Autodesk Fusion 360 part; units mm, degrees
(part 2 of 2)
sketch "Sketch12" plane through (0, 25.45, 0) normal (0, -1, 0) x (1, 0, 0)
  circle A0 centre (0, 0) radius 1.25
  arc A1 (5.596, 0.8992) -> (5.3157, 1.9663) centre (0, 0) ccw
  line L0 (5.3157, 1.9663) -> (5.195, 2.0088)
  arc A2 (5.195, 2.0088) -> (4.3152, 1.9854) centre (4.7857, 0.845) ccw
  arc A3 (4.3152, 1.9854) -> (3.8756, 2.7463) centre (0, 0) ccw
  arc A4 (3.8756, 2.7463) -> (4.2572, 3.2479) centre (3.082, 3.7461) ccw
  line L1 (4.2572, 3.2479) -> (4.3966, 3.5768)
  arc A5 (4.3966, 3.5768) -> (3.6204, 4.3608) centre (0, 0) ccw
  line L2 (3.6204, 4.3608) -> (3.4946, 4.3372)
  arc A6 (3.4946, 4.3372) -> (2.7443, 3.877) centre (3.722, 3.1247) ccw
  arc A7 (2.7443, 3.877) -> (1.9832, 4.3162) centre (0, 0) ccw
  arc A8 (1.9832, 4.3162) -> (2.0629, 4.9414) centre (0.7961, 4.7853) ccw
  line L3 (2.0629, 4.9414) -> (2.0192, 5.2959)
  arc A9 (2.0192, 5.2959) -> (0.955, 5.5867) centre (0, 0) ccw
  line L4 (0.955, 5.5867) -> (0.8578, 5.5034)
  arc A10 (0.8578, 5.5034) -> (0.4382, 4.7297) centre (1.6611, 4.5671) ccw
  arc A11 (0.4382, 4.7297) -> (-0.4406, 4.7295) centre (0, 0) ccw
  arc A12 (-0.4406, 4.7295) -> (-0.6842, 5.3109) centre (-1.7032, 4.5422) ccw
  line L5 (-0.6842, 5.3109) -> (-0.8992, 5.596)
  arc A13 (-0.8992, 5.596) -> (-1.9663, 5.3157) centre (0, 0) ccw
  line L6 (-1.9663, 5.3157) -> (-2.0088, 5.195)
  arc A14 (-2.0088, 5.195) -> (-1.9854, 4.3152) centre (-0.845, 4.7857) ccw
  arc A15 (-1.9854, 4.3152) -> (-2.7463, 3.8756) centre (0, 0) ccw
  arc A16 (-2.7463, 3.8756) -> (-3.2479, 4.2572) centre (-3.7461, 3.082) ccw
  line L7 (-3.2479, 4.2572) -> (-3.5768, 4.3966)
  arc A17 (-3.5768, 4.3966) -> (-4.3608, 3.6204) centre (0, 0) ccw
  line L8 (-4.3608, 3.6204) -> (-4.3372, 3.4946)
  arc A18 (-4.3372, 3.4946) -> (-3.877, 2.7443) centre (-3.1247, 3.722) ccw
  arc A19 (-3.877, 2.7443) -> (-4.3162, 1.9832) centre (0, 0) ccw
  arc A20 (-4.3162, 1.9832) -> (-4.9414, 2.0629) centre (-4.7853, 0.7961) ccw
  line L9 (-4.9414, 2.0629) -> (-5.2959, 2.0192)
  arc A21 (-5.2959, 2.0192) -> (-5.5867, 0.955) centre (0, 0) ccw
  line L10 (-5.5867, 0.955) -> (-5.5034, 0.8578)
  arc A22 (-5.5034, 0.8578) -> (-4.7297, 0.4382) centre (-4.5671, 1.6611) ccw
  arc A23 (-4.7297, 0.4382) -> (-4.7295, -0.4406) centre (0, 0) ccw
  arc A24 (-4.7295, -0.4406) -> (-5.3109, -0.6842) centre (-4.5422, -1.7032) ccw
  line L11 (-5.3109, -0.6842) -> (-5.596, -0.8992)
  arc A25 (-5.596, -0.8992) -> (-5.3157, -1.9663) centre (0, 0) ccw
  line L12 (-5.3157, -1.9663) -> (-5.195, -2.0088)
  arc A26 (-5.195, -2.0088) -> (-4.3152, -1.9854) centre (-4.7857, -0.845) ccw
  arc A27 (-4.3152, -1.9854) -> (-3.8756, -2.7463) centre (0, 0) ccw
  arc A28 (-3.8756, -2.7463) -> (-4.2572, -3.2479) centre (-3.082, -3.7461) ccw
  line L13 (-4.2572, -3.2479) -> (-4.3966, -3.5768)
  arc A29 (-4.3966, -3.5768) -> (-3.6204, -4.3608) centre (0, 0) ccw
  line L14 (-3.6204, -4.3608) -> (-3.4946, -4.3372)
  arc A30 (-3.4946, -4.3372) -> (-2.7443, -3.877) centre (-3.722, -3.1247) ccw
  arc A31 (-2.7443, -3.877) -> (-1.9832, -4.3162) centre (0, 0) ccw
  arc A32 (-1.9832, -4.3162) -> (-2.0629, -4.9414) centre (-0.7961, -4.7853) ccw
  line L15 (-2.0629, -4.9414) -> (-2.0192, -5.2959)
  arc A33 (-2.0192, -5.2959) -> (-0.955, -5.5867) centre (0, 0) ccw
  line L16 (-0.955, -5.5867) -> (-0.8578, -5.5034)
  arc A34 (-0.8578, -5.5034) -> (-0.4382, -4.7297) centre (-1.6611, -4.5671) ccw
  arc A35 (-0.4382, -4.7297) -> (0.4406, -4.7295) centre (0, 0) ccw
  arc A36 (0.4406, -4.7295) -> (0.6842, -5.3109) centre (1.7032, -4.5422) ccw
  line L17 (0.6842, -5.3109) -> (0.8992, -5.596)
  arc A37 (0.8992, -5.596) -> (1.9663, -5.3157) centre (0, 0) ccw
  line L18 (1.9663, -5.3157) -> (2.0088, -5.195)
  arc A38 (2.0088, -5.195) -> (1.9854, -4.3152) centre (0.845, -4.7857) ccw
  arc A39 (1.9854, -4.3152) -> (2.7463, -3.8756) centre (0, 0) ccw
  arc A40 (2.7463, -3.8756) -> (3.2479, -4.2572) centre (3.7461, -3.082) ccw
  line L19 (3.2479, -4.2572) -> (3.5768, -4.3966)
  arc A41 (3.5768, -4.3966) -> (4.3608, -3.6204) centre (0, 0) ccw
  line L20 (4.3608, -3.6204) -> (4.3372, -3.4946)
  arc A42 (4.3372, -3.4946) -> (3.877, -2.7443) centre (3.1247, -3.722) ccw
  arc A43 (3.877, -2.7443) -> (4.3162, -1.9832) centre (0, 0) ccw
  arc A44 (4.3162, -1.9832) -> (4.9414, -2.0629) centre (4.7853, -0.7961) ccw
  line L21 (4.9414, -2.0629) -> (5.2959, -2.0192)
  arc A45 (5.2959, -2.0192) -> (5.5867, -0.955) centre (0, 0) ccw
  line L22 (5.5867, -0.955) -> (5.5034, -0.8578)
  arc A46 (5.5034, -0.8578) -> (4.7297, -0.4382) centre (4.5671, -1.6611) ccw
  arc A47 (4.7297, -0.4382) -> (4.7295, 0.4406) centre (0, 0) ccw
  arc A48 (4.7295, 0.4406) -> (5.3109, 0.6842) centre (4.5422, 1.7032) ccw
  line L23 (5.3109, 0.6842) -> (5.596, 0.8992)
  circle A49 centre (0, 0) radius 3.75
  circle A50 centre (0, 0) radius 1.5
extrude "Extrude13" cut sketch "Sketch12" against normal blind 1 contours A49 bodies 12
sketch "Sketch13" plane through (0, 35.45, 0) normal (0, 1, 0) x (1, 0, 0)
  circle A0 centre (0, 0) radius 32.5
  circle A1 centre (0, 0) radius 31.251
  line L0 (1.3544, -28.9433) -> (0.9515, -29.9849)
  arc A2 (0.9515, -29.9849) -> (0.7328, -31.2424) centre (3.9943, -31.1619) ccw
  arc A3 (2.4106, -31.1579) -> (2.0669, -29.9287) centre (-0.8426, -31.4049) ccw
  line L1 (1.5616, -28.9329) -> (2.0669, -29.9287)
  arc A4 (1.3544, -28.9433) -> (1.5616, -28.9329) centre (0, 0) ccw
  line L2 (2.4106, -31.1579) -> (2.4106, -31.4)
  line L3 (2.4106, -31.4) -> (0.7, -31.4)
  line L4 (0.7, -31.4) -> (0.7328, -31.2424)
  line L5 (4.2295, -28.6646) -> (3.9323, -29.7412)
  arc A5 (3.9323, -29.7412) -> (3.8399, -31.0142) centre (7.0772, -30.6093) ccw
  line L6 (3.823, -31.1743) -> (3.8399, -31.0142)
  line L7 (5.525, -31.004) -> (3.823, -31.1743)
  line L8 (5.5009, -30.763) -> (5.525, -31.004)
  arc A6 (5.5009, -30.763) -> (5.0365, -29.5742) centre (2.2886, -31.3327) ccw
  line L9 (4.4346, -28.6336) -> (5.0365, -29.5742)
  arc A7 (4.2295, -28.6646) -> (4.4346, -28.6336) centre (0, 0) ccw
  line L10 (7.0626, -28.1011) -> (6.8741, -29.2018)
  arc A8 (6.8741, -29.2018) -> (6.9089, -30.4777) centre (10.0897, -29.7526) ccw
  line L11 (6.9079, -30.6387) -> (6.9089, -30.4777)
  line L12 (8.5846, -30.2998) -> (6.9079, -30.6387)
  line L13 (8.5366, -30.0625) -> (8.5846, -30.2998)
  arc A9 (8.5366, -30.0625) -> (7.9562, -28.9258) centre (5.3969, -30.9491) ccw
  line L14 (7.2636, -28.0498) -> (7.9562, -28.9258)
  arc A10 (7.0626, -28.1011) -> (7.2636, -28.0498) centre (0, 0) ccw
  line L15 (9.8255, -27.2582) -> (9.7475, -28.3723)
  arc A11 (9.7475, -28.3723) -> (9.9091, -29.6384) centre (13.002, -28.6001) ccw
  line L16 (9.9242, -29.7987) -> (9.9091, -29.6384)
  line L17 (11.5588, -29.2945) -> (9.9242, -29.7987)
  line L18 (11.4874, -29.0631) -> (11.5588, -29.2945)
  arc A12 (11.4874, -29.0631) -> (10.7967, -27.9898) centre (8.4516, -30.258) ccw
  line L19 (10.0204, -27.1872) -> (10.7967, -27.9898)
  arc A13 (9.8255, -27.2582) -> (10.0204, -27.1872) centre (0, 0) ccw
  line L20 (12.4907, -26.1445) -> (12.524, -27.2608)
  arc A14 (12.524, -27.2608) -> (12.8109, -28.5045) centre (15.785, -27.1634) ccw
  line L21 (12.8419, -28.6624) -> (12.8109, -28.5045)
  line L22 (14.4181, -27.998) -> (12.8419, -28.6624)
  line L23 (14.3241, -27.7749) -> (14.4181, -27.998)
  arc A15 (14.3241, -27.7749) -> (13.5299, -26.7758) centre (11.4224, -29.2661) ccw
  line L24 (12.6775, -26.0544) -> (13.5299, -26.7758)
  arc A16 (12.4907, -26.1445) -> (12.6775, -26.0544) centre (0, 0) ccw
  line L25 (15.0318, -24.7709) -> (15.1761, -25.8783)
  arc A17 (15.1761, -25.8783) -> (15.5854, -27.0873) centre (18.4112, -25.4568) ccw
  line L26 (15.6319, -27.2414) -> (15.5854, -27.0873)
  line L27 (17.1342, -26.4233) -> (15.6319, -27.2414)
  line L28 (17.0184, -26.2107) -> (17.1342, -26.4233)
  arc A18 (17.0184, -26.2107) -> (16.1287, -25.2956) centre (14.2796, -27.9834) ccw
  line L29 (15.2087, -24.6626) -> (16.1287, -25.2956)
  arc A19 (15.0318, -24.7709) -> (15.2087, -24.6626) centre (0, 0) ccw
  line L30 (17.4234, -23.1511) -> (17.6773, -24.2387)
  arc A20 (17.6773, -24.2387) -> (18.205, -25.4009) centre (20.8544, -23.4971) ccw
  line L31 (18.2666, -25.5496) -> (18.205, -25.4009)
  line L32 (19.68, -24.586) -> (18.2666, -25.5496)
  line L33 (19.5436, -24.3859) -> (19.68, -24.586)
  arc A21 (19.5436, -24.3859) -> (18.5672, -23.564) centre (16.9948, -26.4225) ccw
  line L34 (17.5887, -23.0258) -> (18.5672, -23.564)
  arc A22 (17.4234, -23.1511) -> (17.5887, -23.0258) centre (0, 0) ccw
  line L35 (19.642, -21.3013) -> (20.0028, -22.3581)
  arc A23 (20.0028, -22.3581) -> (20.6436, -23.462) centre (23.0903, -21.3039) ccw
  line L36 (20.7198, -23.6038) -> (20.6436, -23.462)
  line L37 (22.0301, -22.5043) -> (20.7198, -23.6038)
  line L38 (21.8745, -22.3188) -> (22.0301, -22.5043)
  arc A24 (21.8745, -22.3188) -> (20.8211, -21.5982) centre (19.5412, -24.5991) ccw
  line L39 (19.794, -21.1601) -> (20.8211, -21.5982)
  arc A25 (19.642, -21.3013) -> (19.794, -21.1601) centre (0, 0) ccw
  line L40 (21.6653, -19.2397) -> (22.1296, -20.2554)
  arc A26 (22.1296, -20.2554) -> (22.8771, -21.29) centre (25.0967, -18.899) ccw
  line L41 (22.967, -21.4235) -> (22.8771, -21.29)
  line L42 (24.1614, -20.199) -> (22.967, -21.4235)
  line L43 (23.988, -20.0299) -> (24.1614, -20.199)
  arc A27 (23.988, -20.0299) -> (22.8681, -19.4177) centre (21.8934, -22.5312) ccw
  line L44 (21.8025, -19.0841) -> (22.8681, -19.4177)
  arc A28 (21.6653, -19.2397) -> (21.8025, -19.0841) centre (0, 0) ccw
  line L45 (23.4733, -16.9869) -> (24.0364, -17.9513)
  arc A29 (24.0364, -17.9513) -> (24.8832, -18.9064) centre (26.8538, -16.3062) ccw
  line L46 (24.986, -19.0303) -> (24.8832, -18.9064)
  line L47 (26.0525, -17.6929) -> (24.986, -19.0303)
  line L48 (25.8632, -17.542) -> (26.0525, -17.6929)
  arc A30 (25.8632, -17.542) -> (24.6879, -17.0443) centre (24.028, -20.2393) ccw
  line L49 (23.5943, -16.8184) -> (24.6879, -17.0443)
  arc A31 (23.4733, -16.9869) -> (23.5943, -16.8184) centre (0, 0) ccw
  line L50 (25.048, -14.5653) -> (25.7043, -15.4689)
  arc A32 (25.7043, -15.4689) -> (26.642, -16.3349) centre (28.3439, -13.5514) ccw
  line L51 (26.7566, -16.4479) -> (26.642, -16.3349)
  line L52 (27.6847, -15.011) -> (26.7566, -16.4479)
  line L53 (27.4813, -14.8797) -> (27.6847, -15.011)
  arc A33 (27.4813, -14.8797) -> (26.2623, -14.5015) centre (25.9238, -17.7464) ccw
  line L54 (25.1516, -14.3856) -> (26.2623, -14.5015)
  arc A34 (25.048, -14.5653) -> (25.1516, -14.3856) centre (0, 0) ccw
  line L55 (26.3738, -11.999) -> (27.1168, -12.8327)
  arc A35 (27.1168, -12.8327) -> (28.1361, -13.601) centre (29.5523, -10.662) ccw
  line L56 (28.2613, -13.7021) -> (28.1361, -13.601)
  line L57 (29.0417, -12.1799) -> (28.2613, -13.7021)
  line L58 (28.8263, -12.0695) -> (29.0417, -12.1799)
  arc A36 (28.8263, -12.0695) -> (27.5757, -11.8145) centre (27.5619, -15.077) ccw
  line L59 (26.459, -11.8098) -> (27.5757, -11.8145)
  arc A37 (26.3738, -11.999) -> (26.459, -11.8098) centre (0, 0) ccw
  line L60 (27.4374, -9.3134) -> (28.2598, -10.069)
  arc A38 (28.2598, -10.069) -> (29.3505, -10.732) centre (30.4671, -7.6665) ccw
  line L61 (29.4852, -10.8201) -> (29.3505, -10.732)
  line L62 (30.1101, -9.2278) -> (29.4852, -10.8201)
  line L63 (29.8847, -9.1393) -> (30.1101, -9.2278)
  arc A39 (29.8847, -9.1393) -> (28.615, -9.0102) centre (28.9261, -12.2578) ccw
  line L64 (27.5034, -9.1167) -> (28.615, -9.0102)
  arc A40 (27.4374, -9.3134) -> (27.5034, -9.1167) centre (0, 0) ccw
  line L65 (28.2284, -6.5352) -> (29.1219, -7.2052)
  arc A41 (29.1219, -7.2052) -> (30.2732, -7.7563) centre (31.079, -4.5949) ccw
  line L66 (30.416, -7.8306) -> (30.2732, -7.7563)
  line L67 (30.8793, -6.1839) -> (30.416, -7.8306)
  line L68 (30.6462, -6.1183) -> (30.8793, -6.1839)
  arc A42 (30.6462, -6.1183) -> (29.3699, -6.1163) centre (30.0029, -9.3168) ccw
  line L69 (28.2744, -6.3329) -> (29.3699, -6.1163)
  arc A43 (28.2284, -6.5352) -> (28.2744, -6.3329) centre (0, 0) ccw
  line L70 (28.7388, -3.6921) -> (29.6946, -4.2697)
  arc A44 (29.6946, -4.2697) -> (30.895, -4.7035) centre (31.3821, -1.4776) ccw
  line L71 (31.0445, -4.7632) -> (30.895, -4.7035)
  line L72 (31.3416, -3.0786) -> (31.0445, -4.7632)
  line L73 (31.1031, -3.0366) -> (31.3416, -3.0786)
  arc A45 (31.1031, -3.0366) -> (29.8329, -3.1616) centre (30.7814, -6.2831) ccw
  line L74 (28.7645, -3.4862) -> (29.8329, -3.1616)
  arc A46 (28.7388, -3.6921) -> (28.7645, -3.4862) centre (0, 0) ccw
  line L75 (28.9636, -0.8123) -> (29.9722, -1.2919)
  arc A47 (29.9722, -1.2919) -> (31.2098, -1.604) centre (31.3733, 1.6544) ccw
  line L76 (31.3645, -1.6485) -> (31.2098, -1.604)
  line L77 (31.4923, 0.0573) -> (31.3645, -1.6485)
  line L78 (31.2509, 0.0754) -> (31.4923, 0.0573)
  arc A48 (31.2509, 0.0754) -> (29.9995, -0.1755) centre (31.2541, -3.1871) ccw
  line L79 (28.9687, -0.6049) -> (29.9995, -0.1755)
  arc A49 (28.9636, -0.8123) -> (28.9687, -0.6049) centre (0, 0) ccw
  line L80 (28.9006, 2.0756) -> (29.9519, 1.6988)
  arc A50 (29.9519, 1.6988) -> (31.2144, 1.5115) centre (31.0526, 4.77) ccw
  line L81 (31.3728, 1.4826) -> (31.2144, 1.5115)
  line L82 (31.3301, 3.1926) -> (31.3728, 1.4826)
  line L83 (31.0881, 3.1866) -> (31.3301, 3.1926)
  arc A51 (31.0881, 3.1866) -> (29.8679, 2.8124) centre (31.4161, -0.0593) ccw
  line L84 (28.885, 2.2825) -> (29.8679, 2.8124)
  arc A52 (28.9006, 2.0756) -> (28.885, 2.2825) centre (0, 0) ccw
  line L85 (28.5503, 4.9428) -> (29.6339, 4.6726)
  arc A53 (29.6339, 4.6726) -> (30.9088, 4.6119) centre (30.4234, 7.8381) ccw
  line L86 (31.0693, 4.599) -> (30.9088, 4.6119)
  line L87 (30.8566, 6.2963) -> (31.0693, 4.599)
  line L88 (30.6163, 6.2661) -> (30.8566, 6.2963)
  arc A54 (30.6163, 6.2661) -> (29.4394, 5.7723) centre (31.2659, 3.069) ccw
  line L89 (28.5142, 5.1471) -> (29.4394, 5.7723)
  arc A55 (28.5503, 4.9428) -> (28.5142, 5.1471) centre (0, 0) ccw
  line L90 (27.9163, 7.761) -> (29.0214, 7.5999)
  arc A56 (29.0214, 7.5999) -> (30.296, 7.6665) centre (29.4918, 10.8283) ccw
  line L91 (30.457, 7.6696) -> (30.296, 7.6665)
  line L92 (30.0763, 9.3373) -> (30.457, 7.6696)
  line L93 (29.8403, 9.2834) -> (30.0763, 9.3373)
  arc A57 (29.8403, 9.2834) -> (28.7184, 8.6748) centre (30.805, 6.1668) ccw
  line L94 (27.86, 7.9606) -> (28.7184, 8.6748)
  arc A58 (27.9163, 7.761) -> (27.86, 7.9606) centre (0, 0) ccw
  line L95 (27.0048, 10.502) -> (28.1205, 10.4518)
  arc A59 (28.1205, 10.4518) -> (29.3821, 10.6449) centre (28.2671, 13.711) ccw
  line L96 (29.542, 10.664) -> (29.3821, 10.6449)
  line L97 (28.9972, 12.2855) -> (29.542, 10.664)
  line L98 (28.7677, 12.2084) -> (28.9972, 12.2855)
  arc A60 (28.7677, 12.2084) -> (27.712, 11.4911) centre (30.0379, 9.2034) ccw
  line L99 (26.9289, 10.695) -> (27.712, 11.4911)
  arc A61 (27.0048, 10.502) -> (26.9289, 10.695) centre (0, 0) ccw
  line L100 (25.825, 13.1386) -> (26.9401, 13.1997)
  arc A62 (26.9401, 13.1997) -> (28.1762, 13.5176) centre (26.7614, 16.4573) ccw
  line L101 (28.3334, 13.5525) -> (28.1762, 13.5176)
  line L102 (27.6298, 15.1117) -> (28.3334, 13.5525)
  line L103 (27.4092, 15.0121) -> (27.6298, 15.1117)
  arc A63 (27.4092, 15.0121) -> (26.4301, 14.1933) centre (28.9723, 12.1484) ccw
  line L104 (25.7302, 13.3232) -> (26.4301, 14.1933)
  arc A64 (25.825, 13.1386) -> (25.7302, 13.3232) centre (0, 0) ccw
  line L105 (24.3884, 15.6446) -> (25.4919, 15.8165)
  arc A65 (25.4919, 15.8165) -> (26.6903, 16.2558) centre (24.9898, 19.0401) ccw
  line L106 (26.8432, 16.3062) -> (26.6903, 16.2558)
  line L107 (25.9879, 17.7876) -> (26.8432, 16.3062)
  line L108 (25.7782, 17.6666) -> (25.9879, 17.7876)
  arc A66 (25.7782, 17.6666) -> (24.8856, 16.7543) centre (27.6187, 14.9728) ccw
  line L109 (24.2758, 15.8188) -> (24.8856, 16.7543)
  arc A67 (24.3884, 15.6446) -> (24.2758, 15.8188) centre (0, 0) ccw
  line L110 (22.7095, 17.9952) -> (23.7904, 18.2761)
  arc A68 (23.7904, 18.2761) -> (24.9391, 18.8326) centre (22.9699, 21.4337) ccw
  line L111 (25.0862, 18.8979) -> (24.9391, 18.8326)
  line L112 (24.0877, 20.2868) -> (25.0862, 18.8979)
  line L113 (23.8911, 20.1455) -> (24.0877, 20.2868)
  arc A69 (23.8911, 20.1455) -> (23.0937, 19.1489) centre (25.9906, 17.6483) ccw
  line L114 (22.5801, 18.1573) -> (23.0937, 19.1489)
  arc A70 (22.7095, 17.9952) -> (22.5801, 18.1573) centre (0, 0) ccw
  line L115 (20.805, 20.1669) -> (21.8525, 20.554)
  arc A71 (21.8525, 20.554) -> (22.9401, 21.2221) centre (20.7216, 23.6142) ccw
  line L116 (23.0799, 21.3018) -> (22.9401, 21.2221)
  line L117 (21.9481, 22.5843) -> (23.0799, 21.3018)
  line L118 (21.7666, 22.4241) -> (21.9481, 22.5843)
  arc A72 (21.7666, 22.4241) -> (21.0724, 21.3531) centre (24.1043, 20.1484) ccw
  line L119 (20.66, 20.3154) -> (21.0724, 21.3531)
  arc A73 (20.805, 20.1669) -> (20.66, 20.3154) centre (0, 0) ccw
  line L120 (18.6936, 22.1382) -> (19.6974, 22.6277)
  arc A74 (19.6974, 22.6277) -> (20.713, 23.4007) centre (18.2674, 25.5601) ccw
  line L121 (20.8443, 23.4939) -> (20.713, 23.4007)
  line L122 (19.5904, 24.6574) -> (20.8443, 23.4939)
  line L123 (19.4257, 24.48) -> (19.5904, 24.6574)
  arc A75 (19.4257, 24.48) -> (18.8416, 23.3451) centre (21.9784, 22.4483) ccw
  line L124 (18.5346, 22.2715) -> (18.8416, 23.3451)
  arc A76 (18.6936, 22.1382) -> (18.5346, 22.2715) centre (0, 0) ccw
  line L125 (16.3964, 23.8895) -> (17.3465, 24.4765)
  arc A77 (17.3465, 24.4765) -> (18.2801, 25.3468) centre (15.6317, 27.2519) ccw
  line L126 (18.4015, 25.4526) -> (18.2801, 25.3468)
  line L127 (17.0379, 26.4855) -> (18.4015, 25.4526)
  line L128 (16.8917, 26.2925) -> (17.0379, 26.4855)
  arc A78 (16.8917, 26.2925) -> (16.4235, 25.1051) centre (19.634, 24.5251) ccw
  line L129 (16.225, 24.0063) -> (16.4235, 25.1051)
  arc A79 (16.3964, 23.8895) -> (16.225, 24.0063) centre (0, 0) ccw
  line L130 (13.9363, 25.4033) -> (14.8233, 26.082)
  arc A80 (14.8233, 26.082) -> (15.6656, 27.041) centre (12.8406, 28.6729) ccw
  line L131 (15.7758, 27.1583) -> (15.6656, 27.041)
  line L132 (14.3161, 28.0503) -> (15.7758, 27.1583)
  line L133 (14.1899, 27.8437) -> (14.3161, 28.0503)
  arc A81 (14.1899, 27.8437) -> (13.8422, 26.6156) centre (17.0945, 26.3582) ccw
  line L134 (13.7541, 25.5025) -> (13.8422, 26.6156)
  arc A82 (13.9363, 25.4033) -> (13.7541, 25.5025) centre (0, 0) ccw
  line L135 (11.3377, 26.6647) -> (12.1527, 27.4283)
  arc A83 (12.1527, 27.4283) -> (12.8953, 28.4664) centre (9.9219, 29.809) ccw
  line L136 (12.9933, 28.5941) -> (12.8953, 28.4664)
  line L137 (11.4521, 29.3363) -> (12.9933, 28.5941)
  line L138 (11.3471, 29.1182) -> (11.4521, 29.3363)
  arc A84 (11.3471, 29.1182) -> (11.1234, 27.8616) centre (14.3852, 27.9292) ccw
  line L139 (11.1465, 26.7452) -> (11.1234, 27.8616)
  arc A85 (11.3377, 26.6647) -> (11.1465, 26.7452) centre (0, 0) ccw
  line L140 (8.6265, 27.6611) -> (9.3613, 28.502)
  arc A86 (9.3613, 28.502) -> (9.9969, 29.6089) centre (6.9046, 30.6487) ccw
  line L141 (10.0816, 29.7458) -> (9.9969, 29.6089)
  line L142 (8.4742, 30.3308) -> (10.0816, 29.7458)
  line L143 (8.3914, 30.1033) -> (8.4742, 30.3308)
  arc A87 (8.3914, 30.1033) -> (8.294, 28.8307) centre (11.5328, 29.2228) ccw
  line L144 (8.4282, 27.7221) -> (8.294, 28.8307)
  arc A88 (8.6265, 27.6611) -> (8.4282, 27.7221) centre (0, 0) ccw
  line L145 (5.8294, 28.3825) -> (6.4769, 29.2925)
  arc A89 (6.4769, 29.2925) -> (6.9991, 30.4571) centre (3.8186, 31.1839) ccw
  line L146 (7.0698, 30.6018) -> (6.9991, 30.4571)
  line L147 (5.4122, 31.0239) -> (7.0698, 30.6018)
  line L148 (5.3524, 30.7892) -> (5.4122, 31.0239)
  arc A90 (5.3524, 30.7892) -> (5.3822, 29.5133) centre (8.5659, 30.2258) ccw
  line L149 (5.6261, 28.4235) -> (5.3822, 29.5133)
  arc A91 (5.8294, 28.3825) -> (5.6261, 28.4235) centre (0, 0) ccw
  line L150 (2.9745, 28.8219) -> (3.5281, 29.7918)
  arc A92 (3.5281, 29.7918) -> (3.9318, 31.0027) centre (0.6947, 31.4092) ccw
  line L151 (3.9877, 31.1536) -> (3.9318, 31.0027)
  line L152 (2.2963, 31.4086) -> (3.9877, 31.1536)
  line L153 (2.2602, 31.1692) -> (2.2963, 31.4086)
  arc A93 (2.2602, 31.1692) -> (2.4169, 29.9025) centre (5.5138, 30.9285) ccw
  line L154 (2.768, 28.8425) -> (2.4169, 29.9025)
  arc A94 (2.9745, 28.8219) -> (2.768, 28.8425) centre (0, 0) ccw
  line L155 (0.09, 28.9749) -> (0.5443, 29.9951)
  arc A95 (0.5443, 29.9951) -> (0.8254, 31.2401) centre (-2.4361, 31.3223) ccw
  line L156 (0.866, 31.3959) -> (0.8254, 31.2401)
  line L157 (-0.8424, 31.4811) -> (0.866, 31.3959)
  line L158 (-0.8545, 31.2393) -> (-0.8424, 31.4811)
  arc A96 (-0.8545, 31.2393) -> (-0.5725, 29.9945) centre (2.4069, 31.3238) ccw
  line L159 (-0.1175, 28.9748) -> (-0.5725, 29.9945)
  arc A97 (0.09, 28.9749) -> (-0.1175, 28.9748) centre (0, 0) ccw
  line L160 (-2.7955, 28.8398) -> (-2.445, 29.9002)
  arc A98 (-2.445, 29.9002) -> (-2.2892, 31.167) centre (-5.5426, 30.9241) ccw
  line L161 (-2.2643, 31.3261) -> (-2.2892, 31.167)
  line L162 (-3.9727, 31.2408) -> (-2.2643, 31.3261)
  line L163 (-3.9607, 30.999) -> (-3.9727, 31.2408)
  arc A99 (-3.9607, 30.999) -> (-3.5561, 29.7885) centre (-0.7239, 31.4078) ccw
  line L164 (-3.0019, 28.8191) -> (-3.5561, 29.7885)
  arc A100 (-2.7955, 28.8398) -> (-3.0019, 28.8191) centre (0, 0) ccw
  line L165 (-5.6531, 28.4182) -> (-5.4099, 29.5082)
  arc A101 (-5.4099, 29.5082) -> (-5.3811, 30.7842) centre (-8.5941, 30.2185) ccw
  line L166 (-5.3721, 30.945) -> (-5.3811, 30.7842)
  line L167 (-7.0636, 30.69) -> (-5.3721, 30.945)
  line L168 (-7.0275, 30.4506) -> (-7.0636, 30.69)
  arc A102 (-7.0275, 30.4506) -> (-6.5044, 29.2864) centre (-3.8475, 31.1797) ccw
  line L169 (-5.8564, 28.377) -> (-6.5044, 29.2864)
  arc A103 (-5.6531, 28.4182) -> (-5.8564, 28.377) centre (0, 0) ccw
  line L170 (-8.4545, 27.7141) -> (-8.3211, 28.8229)
  arc A104 (-8.3211, 28.8229) -> (-8.4195, 30.0955) centre (-11.5602, 29.2127) ccw
  line L171 (-8.4265, 30.2563) -> (-8.4195, 30.0955)
  line L172 (-10.0842, 29.8342) -> (-8.4265, 30.2563)
  line L173 (-10.0245, 29.5996) -> (-10.0842, 29.8342)
  arc A105 (-10.0245, 29.5996) -> (-9.3881, 28.4932) centre (-6.9329, 30.6416) ccw
  line L174 (-8.6527, 27.6529) -> (-9.3881, 28.4932)
  arc A106 (-8.4545, 27.7141) -> (-8.6527, 27.6529) centre (0, 0) ccw
  line L175 (-11.172, 26.7346) -> (-11.1496, 27.8512)
  arc A107 (-11.1496, 27.8512) -> (-11.3742, 29.1076) centre (-14.4114, 27.9165) ccw
  line L176 (-11.3972, 29.2669) -> (-11.3742, 29.1076)
  line L177 (-13.0046, 28.6819) -> (-11.3972, 29.2669)
  line L178 (-12.9218, 28.4544) -> (-13.0046, 28.6819)
  arc A108 (-12.9218, 28.4544) -> (-12.1785, 27.4169) centre (-9.9494, 29.7991) ccw
  line L179 (-11.3631, 26.6539) -> (-12.1785, 27.4169)
  arc A109 (-11.172, 26.7346) -> (-11.3631, 26.6539) centre (0, 0) ccw
  line L180 (-13.7783, 25.4894) -> (-13.8673, 26.6026)
  arc A110 (-13.8673, 26.6026) -> (-14.2158, 27.8305) centre (-17.1194, 26.3428) ccw
  line L181 (-14.2546, 27.9867) -> (-14.2158, 27.8305)
  line L182 (-15.7958, 27.2445) -> (-14.2546, 27.9867)
  line L183 (-15.6907, 27.0264) -> (-15.7958, 27.2445)
  arc A111 (-15.6907, 27.0264) -> (-14.8478, 26.0681) centre (-12.8669, 28.6604) ccw
  line L184 (-13.9605, 25.3901) -> (-14.8478, 26.0681)
  arc A112 (-13.7783, 25.4894) -> (-13.9605, 25.3901) centre (0, 0) ccw
  line L185 (-16.2478, 23.9908) -> (-16.4471, 25.0897)
  arc A113 (-16.4471, 25.0897) -> (-16.9162, 26.2767) centre (-19.6572, 24.5074) ccw
  line L186 (-16.9704, 26.4283) -> (-16.9162, 26.2767)
  line L187 (-18.43, 25.5364) -> (-16.9704, 26.4283)
  line L188 (-18.3037, 25.3298) -> (-18.43, 25.5364)
  arc A114 (-18.3037, 25.3298) -> (-17.3695, 24.4602) centre (-15.6567, 27.2368) ccw
  line L189 (-16.4191, 23.8739) -> (-17.3695, 24.4602)
  arc A115 (-16.2478, 23.9908) -> (-16.4191, 23.8739) centre (0, 0) ccw
  line L190 (-18.5558, 22.2539) -> (-18.8635, 23.3274)
  arc A116 (-18.8635, 23.3274) -> (-19.4485, 24.4619) centre (-21.9997, 22.4284) ccw
  line L191 (-19.5175, 24.6073) -> (-19.4485, 24.4619)
  line L192 (-20.881, 23.5744) -> (-19.5175, 24.6073)
  line L193 (-20.7348, 23.3815) -> (-20.881, 23.5744)
  arc A117 (-20.7348, 23.3815) -> (-19.7187, 22.6092) centre (-18.2908, 25.5426) ccw
  line L194 (-18.7146, 22.1204) -> (-19.7187, 22.6092)
  arc A118 (-18.5558, 22.2539) -> (-18.7146, 22.1204) centre (0, 0) ccw
  line L195 (-20.6793, 20.2957) -> (-21.0924, 21.3333)
  arc A119 (-21.0924, 21.3333) -> (-21.7874, 22.4039) centre (-24.1235, 20.1265) ccw
  line L196 (-21.8706, 22.5417) -> (-21.7874, 22.4039)
  line L197 (-23.1245, 21.3782) -> (-21.8706, 22.5417)
  line L198 (-22.9598, 21.2007) -> (-23.1245, 21.3782)
  arc A120 (-22.9598, 21.2007) -> (-21.8718, 20.5335) centre (-20.7431, 23.5945) ccw
  line L199 (-20.8241, 20.1471) -> (-21.8718, 20.5335)
  arc A121 (-20.6793, 20.2957) -> (-20.8241, 20.1471) centre (0, 0) ccw
  line L200 (-22.5974, 18.1359) -> (-23.1117, 19.1271)
  arc A122 (-23.1117, 19.1271) -> (-23.9099, 20.1232) centre (-26.0076, 17.6245) ccw
  line L201 (-24.0063, 20.2521) -> (-23.9099, 20.1232)
  line L202 (-25.1382, 18.9695) -> (-24.0063, 20.2521)
  line L203 (-24.9566, 18.8093) -> (-25.1382, 18.9695)
  arc A123 (-24.9566, 18.8093) -> (-23.8076, 18.2537) centre (-22.9893, 21.4119) ccw
  line L204 (-22.7266, 17.9736) -> (-23.8076, 18.2537)
  arc A124 (-22.5974, 18.1359) -> (-22.7266, 17.9736) centre (0, 0) ccw
  line L205 (-24.2908, 15.7958) -> (-24.9013, 16.7309)
  arc A125 (-24.9013, 16.7309) -> (-25.7947, 17.6426) centre (-27.6332, 14.9474) ccw
  line L206 (-25.9035, 17.7612) -> (-25.7947, 17.6426)
  line L207 (-26.902, 16.3723) -> (-25.9035, 17.7612)
  line L208 (-26.7054, 16.231) -> (-26.902, 16.3723)
  arc A126 (-26.7054, 16.231) -> (-25.5068, 15.7925) centre (-25.007, 19.0165) ccw
  line L209 (-24.4033, 15.6214) -> (-25.5068, 15.7925)
  arc A127 (-24.2908, 15.7958) -> (-24.4033, 15.6214) centre (0, 0) ccw
  line L210 (-25.7429, 13.2987) -> (-26.4435, 14.1684)
  arc A128 (-26.4435, 14.1684) -> (-27.4231, 14.9866) centre (-28.9841, 12.1218) ccw
  line L211 (-27.5432, 15.0938) -> (-27.4231, 14.9866)
  line L212 (-28.3985, 13.6124) -> (-27.5432, 15.0938)
  line L213 (-28.1888, 13.4913) -> (-28.3985, 13.6124)
  arc A129 (-28.1888, 13.4913) -> (-26.9525, 13.1744) centre (-26.7761, 16.4321) ccw
  line L214 (-25.8374, 13.114) -> (-26.9525, 13.1744)
  arc A130 (-25.7429, 13.2987) -> (-25.8374, 13.114) centre (0, 0) ccw
  line L215 (-26.9391, 10.6694) -> (-27.7228, 11.4651)
  arc A131 (-27.7228, 11.4651) -> (-28.779, 12.1816) centre (-30.0471, 9.1757) ccw
  line L216 (-28.9092, 12.2764) -> (-28.779, 12.1816)
  line L217 (-29.6127, 10.7172) -> (-28.9092, 12.2764)
  line L218 (-29.392, 10.6176) -> (-29.6127, 10.7172)
  arc A132 (-29.392, 10.6176) -> (-28.1303, 10.4253) centre (-28.2792, 13.6844) ccw
  line L219 (-27.0148, 10.4763) -> (-28.1303, 10.4253)
  arc A133 (-26.9391, 10.6694) -> (-27.0148, 10.4763) centre (0, 0) ccw
  line L220 (-27.8675, 7.9342) -> (-28.7266, 8.6478)
  arc A134 (-28.7266, 8.6478) -> (-29.8489, 9.2556) centre (-30.8113, 6.1383) ccw
  line L221 (-29.9879, 9.3369) -> (-29.8489, 9.2556)
  line L222 (-30.5327, 7.7154) -> (-29.9879, 9.3369)
  line L223 (-30.3032, 7.6383) -> (-30.5327, 7.7154)
  arc A135 (-30.3032, 7.6383) -> (-29.0285, 7.5726) centre (-29.5012, 10.8007) ccw
  line L224 (-27.9236, 7.7344) -> (-29.0285, 7.5726)
  arc A136 (-27.8675, 7.9342) -> (-27.9236, 7.7344) centre (0, 0) ccw
  line L225 (-28.519, 5.12) -> (-29.4449, 5.7446)
  arc A137 (-29.4449, 5.7446) -> (-30.6222, 6.2376) centre (-31.2694, 3.04) ccw
  line L226 (-30.7685, 6.3047) -> (-30.6222, 6.2376)
  line L227 (-31.1491, 4.637) -> (-30.7685, 6.3047)
  line L228 (-30.9131, 4.5832) -> (-31.1491, 4.637)
  arc A138 (-30.9131, 4.5832) -> (-29.6383, 4.6447) centre (-30.43, 7.8097) ccw
  line L229 (-28.555, 4.9157) -> (-29.6383, 4.6447)
  arc A139 (-28.519, 5.12) -> (-28.555, 4.9157) centre (0, 0) ccw
  line L230 (-28.8871, 2.255) -> (-29.8705, 2.7843)
  arc A140 (-29.8705, 2.7843) -> (-31.0911, 3.1577) centre (-31.4167, -0.0885) ccw
  line L231 (-31.2434, 3.2098) -> (-31.0911, 3.1577)
  line L232 (-31.456, 1.5125) -> (-31.2434, 3.2098)
  line L233 (-31.2158, 1.4824) -> (-31.456, 1.5125)
  arc A141 (-31.2158, 1.4824) -> (-29.9534, 1.6706) centre (-31.0564, 4.741) ccw
  line L234 (-28.9025, 2.0481) -> (-29.9534, 1.6706)
  arc A142 (-28.8871, 2.255) -> (-28.9025, 2.0481) centre (0, 0) ccw
  line L235 (-28.9681, -0.6324) -> (-29.9993, -0.2037)
  arc A143 (-29.9993, -0.2037) -> (-31.251, 0.0463) centre (-31.2518, -3.2162) ccw
  line L236 (-31.4077, 0.083) -> (-31.251, 0.0463)
  line L237 (-31.4503, -1.627) -> (-31.4077, 0.083)
  line L238 (-31.2083, -1.633) -> (-31.4503, -1.627)
  arc A144 (-31.2083, -1.633) -> (-29.9709, -1.3201) centre (-31.3741, 1.6252) ccw
  line L239 (-28.9628, -0.8398) -> (-29.9709, -1.3201)
  arc A145 (-28.9681, -0.6324) -> (-28.9628, -0.8398) centre (0, 0) ccw
  line L240 (-28.7612, -3.5136) -> (-29.83, -3.1896)
  arc A146 (-29.83, -3.1896) -> (-31.1003, -3.0655) centre (-30.7763, -6.3119) ccw
  line L241 (-31.2599, -3.0446) -> (-31.1003, -3.0655)
  line L242 (-31.1321, -4.7504) -> (-31.2599, -3.0446)
  line L243 (-30.8906, -4.7323) -> (-31.1321, -4.7504)
  arc A147 (-30.8906, -4.7323) -> (-29.6906, -4.2977) centre (-31.38, -1.5067) ccw
  line L244 (-28.7353, -3.7194) -> (-29.6906, -4.2977)
  arc A148 (-28.7612, -3.5136) -> (-28.7353, -3.7194) centre (0, 0) ccw
  line L245 (-28.2684, -6.3598) -> (-29.3641, -6.1439)
  arc A149 (-29.3641, -6.1439) -> (-30.6405, -6.1469) centre (-29.9949, -9.3448) ccw
  line L246 (-30.8014, -6.1419) -> (-30.6405, -6.1469)
  line L247 (-30.5044, -7.8265) -> (-30.8014, -6.1419)
  line L248 (-30.2659, -7.7845) -> (-30.5044, -7.8265)
  arc A150 (-30.2659, -7.7845) -> (-29.1151, -7.2325) centre (-31.0741, -4.6236) ccw
  line L249 (-28.2222, -6.562) -> (-29.1151, -7.2325)
  arc A151 (-28.2684, -6.3598) -> (-28.2222, -6.562) centre (0, 0) ccw
  line L250 (-27.4947, -9.1428) -> (-28.6065, -9.0371)
  arc A152 (-28.6065, -9.0371) -> (-29.8762, -9.1671) centre (-28.9154, -12.2849) ccw
  line L251 (-30.0368, -9.1782) -> (-29.8762, -9.1671)
  line L252 (-29.5735, -10.8249) -> (-30.0368, -9.1782)
  line L253 (-29.3405, -10.7593) -> (-29.5735, -10.8249)
  arc A153 (-29.3405, -10.7593) -> (-28.2503, -10.0955) centre (-30.4593, -7.6946) ccw
  line L254 (-27.4285, -9.3395) -> (-28.2503, -10.0955)
  arc A154 (-27.4947, -9.1428) -> (-27.4285, -9.3395) centre (0, 0) ccw
  line L255 (-26.4478, -11.835) -> (-27.5645, -11.8405)
  arc A155 (-27.5645, -11.8405) -> (-28.815, -12.0963) centre (-27.5485, -15.1029) ccw
  line L256 (-28.9737, -12.1233) -> (-28.815, -12.0963)
  line L257 (-28.3488, -13.7156) -> (-28.9737, -12.1233)
  line L258 (-28.1234, -13.6272) -> (-28.3488, -13.7156)
  arc A156 (-28.1234, -13.6272) -> (-27.1047, -12.8582) centre (-29.5418, -10.6892) ccw
  line L259 (-26.3623, -12.024) -> (-27.1047, -12.8582)
  arc A157 (-26.4478, -11.835) -> (-26.3623, -12.024) centre (0, 0) ccw
  line L260 (-25.1379, -14.4095) -> (-26.2486, -14.5262)
  arc A158 (-26.2486, -14.5262) -> (-27.4674, -14.9052) centre (-25.9078, -17.7708) ccw
  line L261 (-27.6226, -14.9479) -> (-27.4674, -14.9052)
  line L262 (-26.8422, -16.4701) -> (-27.6226, -14.9479)
  line L263 (-26.6268, -16.3597) -> (-26.8422, -16.4701)
  arc A159 (-26.6268, -16.3597) -> (-25.6898, -15.4931) centre (-28.3307, -13.5775) ccw
  line L264 (-25.0341, -14.5891) -> (-25.6898, -15.4931)
  arc A160 (-25.1379, -14.4095) -> (-25.0341, -14.5891) centre (0, 0) ccw
  line L265 (-23.5783, -16.8409) -> (-24.6718, -17.0675)
  arc A161 (-24.6718, -17.0675) -> (-25.8468, -17.566) centre (-24.0097, -20.2621) ccw
  line L266 (-25.997, -17.624) -> (-25.8468, -17.566)
  line L267 (-25.069, -19.0609) -> (-25.997, -17.624)
  line L268 (-24.8656, -18.9295) -> (-25.069, -19.0609)
  arc A162 (-24.8656, -18.9295) -> (-24.0195, -17.9739) centre (-26.838, -16.3308) ccw
  line L269 (-23.4571, -17.0092) -> (-24.0195, -17.9739)
  arc A163 (-23.5783, -16.8409) -> (-23.4571, -17.0092) centre (0, 0) ccw
  line L270 (-21.7843, -19.1048) -> (-22.8499, -19.4392)
  arc A164 (-22.8499, -19.4392) -> (-23.9694, -20.0523) centre (-21.8729, -22.552) ccw
  line L271 (-24.1131, -20.1249) -> (-23.9694, -20.0523)
  line L272 (-23.0465, -21.4622) -> (-24.1131, -20.1249)
  line L273 (-22.8573, -21.3113) -> (-23.0465, -21.4622)
  arc A165 (-22.8573, -21.3113) -> (-22.1105, -20.2762) centre (-25.0786, -18.9219) ccw
  line L274 (-21.647, -19.2603) -> (-22.1105, -20.2762)
  arc A166 (-21.7843, -19.1048) -> (-21.647, -19.2603) centre (0, 0) ccw
  line L275 (-19.7739, -21.1789) -> (-20.8008, -21.6177)
  arc A167 (-20.8008, -21.6177) -> (-21.8537, -22.3392) centre (-19.5188, -24.6178) ccw
  line L276 (-21.9895, -22.4257) -> (-21.8537, -22.3392)
  line L277 (-20.7951, -23.6503) -> (-21.9895, -22.4257)
  line L278 (-20.6218, -23.4812) -> (-20.7951, -23.6503)
  arc A168 (-20.6218, -23.4812) -> (-19.9818, -22.3769) centre (-23.07, -21.3249) ccw
  line L279 (-19.6217, -21.3199) -> (-19.9818, -22.3769)
  arc A169 (-19.7739, -21.1789) -> (-19.6217, -21.3199) centre (0, 0) ccw
  line L280 (-17.5669, -23.0425) -> (-18.545, -23.5814)
  arc A170 (-18.545, -23.5814) -> (-19.5209, -24.4041) centre (-16.9707, -26.4389) ccw
  line L281 (-19.6473, -24.5037) -> (-19.5209, -24.4041)
  line L282 (-18.3369, -25.6033) -> (-19.6473, -24.5037)
  line L283 (-18.1813, -25.4178) -> (-18.3369, -25.6033)
  arc A171 (-18.1813, -25.4178) -> (-17.6545, -24.2553) centre (-20.8321, -23.5159) ccw
  line L284 (-17.4014, -23.1677) -> (-17.6545, -24.2553)
  arc A172 (-17.5669, -23.0425) -> (-17.4014, -23.1677) centre (0, 0) ccw
  line L285 (-15.1853, -24.6771) -> (-16.1049, -25.3107)
  arc A173 (-16.1049, -25.3107) -> (-16.994, -26.2265) centre (-14.2539, -27.9972) ccw
  line L286 (-17.1099, -26.3382) -> (-16.994, -26.2265)
  line L287 (-15.6965, -27.3018) -> (-17.1099, -26.3382)
  line L288 (-15.5602, -27.1018) -> (-15.6965, -27.3018)
  arc A174 (-15.5602, -27.1018) -> (-15.1517, -25.8926) centre (-18.3871, -25.4733) ccw
  line L289 (-15.0082, -24.7852) -> (-15.1517, -25.8926)
  arc A175 (-15.1853, -24.6771) -> (-15.0082, -24.7852) centre (0, 0) ccw
  line L290 (-12.6528, -26.0664) -> (-13.5047, -26.7885)
  arc A176 (-13.5047, -26.7885) -> (-14.2982, -27.7882) centre (-11.3954, -29.2773) ccw
  line L291 (-14.4024, -27.9109) -> (-14.2982, -27.7882)
  line L292 (-12.9002, -28.729) -> (-14.4024, -27.9109)
  line L293 (-12.7844, -28.5164) -> (-12.9002, -28.729)
  arc A177 (-12.7844, -28.5164) -> (-12.4984, -27.2725) centre (-15.7594, -27.1775) ccw
  line L294 (-12.4658, -26.1563) -> (-12.4984, -27.2725)
  arc A178 (-12.6528, -26.0664) -> (-12.4658, -26.1563) centre (0, 0) ccw
  line L295 (-9.9945, -27.1967) -> (-10.7704, -28)
  arc A179 (-10.7704, -28) -> (-11.4604, -29.0738) centre (-8.4237, -30.2665) ccw
  line L296 (-11.5518, -29.2063) -> (-11.4604, -29.0738)
  line L297 (-9.9756, -29.8707) -> (-11.5518, -29.2063)
  line L298 (-9.8815, -29.6476) -> (-9.9756, -29.8707)
  arc A180 (-9.8815, -29.6476) -> (-9.7208, -28.3814) centre (-12.9751, -28.6116) ccw
  line L299 (-9.7995, -27.2676) -> (-9.7208, -28.3814)
  arc A181 (-9.9945, -27.1967) -> (-9.7995, -27.2676) centre (0, 0) ccw
  line L300 (-7.2369, -28.0567) -> (-7.9289, -28.9332)
  arc A182 (-7.9289, -28.9332) -> (-8.5086, -30.0704) centre (-5.3683, -30.9548) ccw
  line L301 (-8.5864, -30.2113) -> (-8.5086, -30.0704)
  line L302 (-6.9518, -30.7155) -> (-8.5864, -30.2113)
  line L303 (-6.8805, -30.4842) -> (-6.9518, -30.7155)
  arc A183 (-6.8805, -30.4842) -> (-6.8466, -29.2083) centre (-10.0619, -29.7613) ccw
  line L304 (-7.0359, -28.1078) -> (-6.8466, -29.2083)
  arc A184 (-7.2369, -28.0567) -> (-7.0359, -28.1078) centre (0, 0) ccw
  line L305 (-4.4074, -28.6378) -> (-5.0087, -29.5789)
  arc A185 (-5.0087, -29.5789) -> (-5.4723, -30.7682) centre (-2.2595, -31.3355) ccw
  line L306 (-5.5357, -30.9161) -> (-5.4723, -30.7682)
  line L307 (-3.859, -31.2551) -> (-5.5357, -30.9161)
  line L308 (-3.811, -31.0178) -> (-3.859, -31.2551)
  arc A186 (-3.811, -31.0178) -> (-3.9044, -29.7448) centre (-7.0486, -30.6152) ccw
  line L309 (-4.2023, -28.6686) -> (-3.9044, -29.7448)
  arc A187 (-4.4074, -28.6378) -> (-4.2023, -28.6686) centre (0, 0) ccw
  line L310 (-1.5341, -28.9344) -> (-2.0387, -29.9306)
  arc A188 (-2.0387, -29.9306) -> (-2.3816, -31.1601) centre (0.8717, -31.4048) ccw
  line L311 (-2.4299, -31.3137) -> (-2.3816, -31.1601)
  line L312 (-0.7278, -31.484) -> (-2.4299, -31.3137)
  line L313 (-0.7037, -31.2431) -> (-0.7278, -31.484)
  arc A189 (-0.7037, -31.2431) -> (-0.9233, -29.9858) centre (-3.9653, -31.1649) ccw
  line L314 (-1.3269, -28.9446) -> (-0.9233, -29.9858)
  arc A190 (-1.5341, -28.9344) -> (-1.3269, -28.9446) centre (0, 0) ccw
  dimension "d82" = 65
  dimension "d83" = 62.502
  dimension "d85" = 57.95
  dimension "d87" = 360
  constraint coincident A0.centre A1.centre
  constraint concentric A0 A1
  constraint concentric A1 A4
  constraint coincident A1 A2.end
  constraint tangent L0 A2
  constraint vertical L2
  constraint perpendicular L2 L3
  measures "d82" diameter of A0
  measures "d83" diameter of A1
  measures "d85" diameter of A4
extrude "Extrude14" add sketch "Sketch13" sketch "Sketch11" against normal blind 10 separate body contours A0 | A1 L75 A47 A48 L79 A49 | A1 L76 L77 L78 | A1 L80 A50 A51 L84 A52 | A1 L81 L82 L83 | A1 L71 L72 L73 | A1 L70 A44 A45 L74 A46 | A1 L85 A53 A54 L89 A55 | A1 L86 L87 L88 | A1 L66 L67 L68 | A1 L65 A41 A42 L69 A43 | A1 L90 A56 A57 L94 A58 | A1 L91 L92 L93 | A1 L61 L62 L63 | A1 L60 A38 A39 L64 A40 | A1 L95 A59 A60 L99 A61 | A1 L96 L97 L98 | A1 L56 L57 L58 | A1 L55 A35 A36 L59 A37 | A1 L100 A62 A63 L104 A64 | A1 L101 L102 L103 | A1 L51 L52 L53 | A1 L50 A32 A33 L54 A34 | A1 L105 A65 A66 L109 A67 | A1 L106 L107 L108 | A1 L46 L47 L48 | A1 L45 A29 A30 L49 A31 | A1 L110 A68 A69 L114 A70 | A1 L111 L112 L113 | A1 L41 L42 L43 | A1 L40 A26 A27 L44 A28 | A1 L115 A71 A72 L119 A73 | A1 L116 L117 L118 | A1 L36 L37 L38 | A1 L35 A23 A24 L39 A25 | A1 L120 A74 A75 L124 A76 | A1 L121 L122 L123 | A1 L31 L32 L33 | A1 L30 A20 A21 L34 A22 | A1 L125 A77 A78 L129 A79 | A1 L126 L127 L128 | A1 L26 L27 L28 | A1 L25 A17 A18 L29 A19 | A1 L130 A80 A81 L134 A82 | A1 L131 L132 L133 | A1 L21 L22 L23 | A1 L20 A14 A15 L24 A16 | A1 L135 A83 A84 L139 A85 | A1 L136 L137 L138 | A1 L16 L17 L18 | A1 L15 A11 A12 L19 A13 | A1 L140 A86 A87 L144 A88 | A1 L141 L142 L143 | A1 L11 L12 L13 | A1 L10 A8 A9 L14 A10 | A1 L145 A89 A90 L149 A91 | A1 L146 L147 L148 | A1 L6 L7 L8 | A1 L5 A5 A6 L9 A7 | A1 L150 A92 A93 L154 A94 | A1 L151 L152 L153 | A1 L2 L3 L4 | A1 L0 A2 A3 L1 A4 | A1 L155 A95 A96 L159 A97 | A1 L156 L157 L158 | A1 L311 L312 L313 | A1 L310 A188 A189 L314 A190 | A1 L160 A98 A99 L164 A100 | A1 L161 L162 L163 | A1 L306 L307 L308 | A1 L305 A185 A186 L309 A187 | A1 L165 A101 A102 L169 A103 | A1 L166 L167 L168 | A1 L301 L302 L303 | A1 L300 A182 A183 L304 A184 | A1 L170 A104 A105 L174 A106 | A1 L171 L172 L173 | A1 L296 L297 L298 | A1 L295 A179 A180 L299 A181 | A1 L175 A107 A108 L179 A109 | A1 L176 L177 L178 | A1 L291 L292 L293 | A1 L290 A176 A177 L294 A178 | A1 L180 A110 A111 L184 A112 | A1 L181 L182 L183 | A1 L286 L287 L288 | A1 L285 A173 A174 L289 A175 | A1 L185 A113 A114 L189 A115 | A1 L186 L187 L188 | A1 L281 L282 L283 | A1 L280 A170 A171 L284 A172 | A1 L190 A116 A117 L194 A118 | A1 L191 L192 L193 | A1 L276 L277 L278 | A1 L275 A167 A168 L279 A169 | A1 L195 A119 A120 L199 A121 | A1 L196 L197 L198 | A1 L271 L272 L273 | A1 L270 A164 A165 L274 A166 | A1 L200 A122 A123 L204 A124 | A1 L201 L202 L203 | A1 L266 L267 L268 | A1 L265 A161 A162 L269 A163 | A1 L205 A125 A126 L209 A127 | A1 L206 L207 L208 | A1 L261 L262 L263 | A1 L260 A158 A159 L264 A160 | A1 L210 A128 A129 L214 A130 | A1 L211 L212 L213 | A1 L256 L257 L258 | A1 L255 A155 A156 L259 A157 | A1 L215 A131 A132 L219 A133 | A1 L216 L217 L218 | A1 L251 L252 L253 | A1 L250 A152 A153 L254 A154 | A1 L220 A134 A135 L224 A136 | A1 L221 L222 L223 | A1 L246 L247 L248 | A1 L245 A149 A150 L249 A151 | A1 L225 A137 A138 L229 A139 | A1 L226 L227 L228 | A1 L241 L242 L243 | A1 L240 A146 A147 L244 A148 | A1 L230 A140 A141 L234 A142 | A1 L231 L232 L233 | A1 L236 L237 L238 | A1 L235 A143 A144 L239 A145 of sketch 2 contours A0 | A1 L0 A2 A3 A4 L1 A5 L2 A6 A7 A8 L3 A9 L4 A10 A11 A12 L5 A13 L6 A14 A15 A16 L7 A17 L8 A18 A19 A20 L9 A21 L10 A22 A23 A24 L11 A25 L12 A26 A27 A28 L13 A29 L14 A30 A31 A32 L15 A33 L16 A34 A35 A36 L17 A37 L18 A38 A39 A40 L19 A41 L20 A42 A43 A44 L21 A45 L22 A46 A47 A48 L23 | A49 | A50 makes body 13 at (32.4596, 28.7833, 1.62) makes body 14 at (2.3672, 35.45, 0.286)
hidden bodies 14
equation "d45 = 1.5 mm + 22.5 mm"
named bodies: "Carrier scale", "planet gear", "planet gear 2", "planet gear 3", "PG-1ROD", "PG-1ROD (1)", "PG-1ROD (2)", "screw hold", "screw hold (1)", "screw hold (2)", "sun gear"
